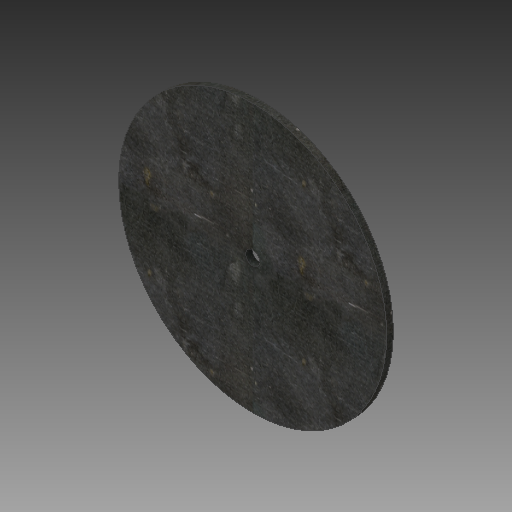
# Autodesk Inventor part: saw blade
Saved by Autodesk Inventor 2019 (Build 230136000, 136)
## iProperties
Created: 2017-12-10
Part Number: saw blade
Material: Steel
Document SubType Name: Modeling
Designer: rk_fe
Density: 7.85 g/cm^3
Appearance: Plate
Author: rk_fe
Autodesk Inventor part; units mm, degrees
ref_plane "YZ Plane" through (0, 0, 0) normal (1, 0, 0) x (0, 1, 0)
ref_plane "XZ Plane" through (0, 0, 0) normal (0, 1, 0) x (-1, 0, 0)
ref_plane "XY Plane" through (0, 0, 0) normal (0, 0, 1) x (1, 0, 0)
sketch "Sketch1" plane through (0, 0, 0) normal (0, 0, 1) x (1, 0, 0)
  circle A0 centre (0, 0) radius 152.4
  circle A1 centre (0, 0) radius 7.9375
  dimension "d0" = 304.8
  dimension "d1" = 15.875
  constraints: 2 centre point, 2 coincident
  measures "d0" diameter of A0
  measures "d1" diameter of A1
extrude "Extrusion1" add sketch "Sketch1" along normal blind 7.62
body "Solid1"
